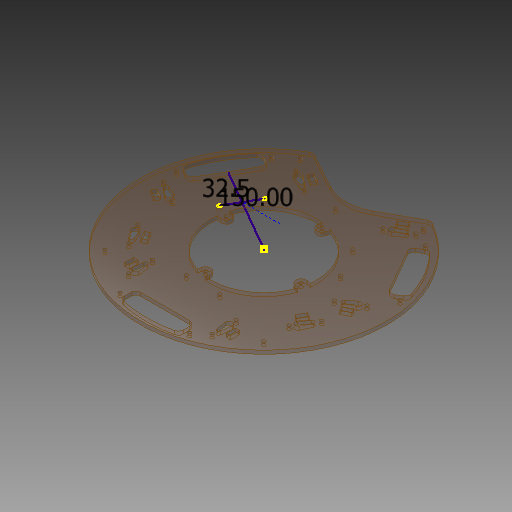
# Autodesk Inventor part: Base Plate
Saved by Autodesk Inventor 2018 (Build 220112000, 112)
## iProperties
Created: 2018-06-09
Part Number: Base Plate
Material: Polycarbonate, Smoke
Document SubType Name: Modeling
Designer: matth
Density: 1.2 g/cm^3
Appearance: Polycarbonate - Smoked
Mass: 68.8763 g
Surface Area: 521.491 cm^2
Volume: 68.8763 cm^3
Author: matth
Autodesk Inventor part; units mm, degrees
ref_plane "YZ Plane" through (0, 0, 0) normal (1, 0, 0) x (0, 1, 0)
ref_plane "XZ Plane" through (0, 0, 0) normal (0, 1, 0) x (-1, 0, 0)
ref_plane "XY Plane" through (0, 0, 0) normal (0, 0, 1) x (1, 0, 0)
sketch "Sketch1" plane through (0, 0, 0) normal (0, 1, 0) x (-1, 0, 0)
  circle A0 centre (0, 0) radius 105
  dimension "d0" = 210
  constraints: 1 centre point, 1 coincident
  measures "d0" diameter of A0
extrude "Blank Disk" add sketch "Sketch1" along normal blind 3
sketch "Sketch2" plane through (0, 3, 0) normal (0, 1, 0) x (1, 0, 0)
  line L0 (0, 0) -> (90.9327, 52.5)
  line L1 (0, 0) -> (105, 0) construction
  line L2 (0, 0) -> (-90.9327, 52.5)
  circle A0 centre (0, 0) radius 105 projected
  line L3 (0, 0) -> (0, -105)
  line L4 (90.9327, 52.5) -> (78.4327, 74.1506)
  line L5 (90.9327, 52.5) -> (103.4327, 30.8494)
  circle A1 centre (0, 0) radius 100
  line L6 (78.4327, 74.1506) -> (71.3525, 70.0629)
  line L7 (103.4327, 30.8494) -> (96.3525, 26.7617)
  line L8 (96.3525, 26.7617) -> (85.0942, 20.2617)
  line L9 (85.0942, 20.2617) -> (60.0942, 63.5629)
  line L10 (60.0942, 63.5629) -> (71.3525, 70.0629)
  arc A2 (96.3525, 26.7617) -> (71.3525, 70.0629) centre (0, 0) ccw
  line L11 (-90.9327, 52.5) -> (-78.4327, 74.1506)
  line L12 (-78.4327, 74.1506) -> (-103.4327, 30.8494)
  line L13 (-103.4327, 30.8494) -> (-96.3525, 26.7617)
  line L14 (-96.3525, 26.7617) -> (-85.0942, 20.2617)
  line L15 (-85.0942, 20.2617) -> (-60.0942, 63.5629)
  line L16 (-60.0942, 63.5629) -> (-71.3525, 70.0629)
  arc A3 (-71.3525, 70.0629) -> (-96.3525, 26.7617) centre (0, 0) ccw
  line L17 (0, -105) -> (25, -105)
  line L18 (25, -105) -> (25, -96.8246)
  line L19 (25, -96.8246) -> (25, -83.8246)
  line L20 (25, -83.8246) -> (-25, -83.8246)
  line L21 (-25, -83.8246) -> (-25, -96.8246)
  arc A4 (-25, -96.8246) -> (25, -96.8246) centre (0, 0) ccw
  dimension "d3" = 105
  dimension "d4" = 30
  dimension "d5" = 25
  dimension "d6" = 25
  dimension "d7" = 200
  dimension "d8" = 13
  dimension "d9" = 25
  dimension "d10" = 50
  dimension "d11" = 13
  dimension "d12" = 25
  dimension "d13" = 13
  dimension "d14" = 50
  constraints: 44 end point, 14 point on circle, 7 perpendicular, 5 point on line, 4 centre point, 2 concentric, 2 horizontal, 1 coincident, 1 equal length, 1 parallel, 1 vertical
  measures "d3" distance of L0.start L0.end
  measures "d4" angle of L1 L0
  measures "d5" distance of L0.end L4.end
  measures "d6" distance of L0.end L5.end
  measures "d7" diameter of A1
  measures "d8" distance of L7.end L8.end
  measures "d9" distance of L2.end L11.end
  measures "d10" distance of L11.end L12.end
  measures "d11" distance of L13.end L14.end
  measures "d12" distance of L3.end L17.end
  measures "d13" distance of L18.end L19.end
  measures "d14" distance of L19.end L20.end
extrude "Wheel Holes" cut sketch "Sketch2" against normal blind 3 contours L9 L10 A1 L0 | L0 A1 L8 L9 | L15 L14 A1 L2 | L2 A1 L16 L15 | L20 L19 A1 L3 | L3 A1 L21 L20
sketch "Sketch3" plane through (0, 3, 0) normal (0, 1, 0) x (1, 0, 0)
  line L0 (-60.0942, 63.5629) -> (-71.3525, 70.0629) projected
  line L1 (-96.3525, 26.7617) -> (-85.0942, 20.2617) projected
  line L2 (-71.3525, 70.0629) -> (-96.3525, 26.7617)
  line L3 (-83.8525, 48.4123) -> (-80.3884, 46.4123)
  line L4 (-80.3884, 46.4123) -> (-77.7904, 44.9123)
  line L5 (-77.7904, 44.9123) -> (-72.5942, 41.9123)
  line L6 (-72.5942, 41.9123) -> (-44.6649, 25.7873)
  line L7 (-60.0942, 63.5629) -> (-85.0942, 20.2617) projected
  line L8 (-72.5942, 41.9123) -> (-40.3442, 41.9123) construction
  line L9 (-44.6649, 25.7873) -> (-37.6149, 37.9983)
  line L10 (-37.6149, 37.9983) -> (-51.7149, 13.5763)
  circle A0 centre (-37.6149, 37.9983) radius 1.25
  circle A1 centre (-51.7149, 13.5763) radius 1.25
  line L11 (-72.5942, 41.9123) -> (-13.7045, 7.9123)
  line L12 (-13.7045, 7.9123) -> (-7.4545, 18.7376)
  line L13 (-13.7045, 7.9123) -> (-19.9545, -2.913)
  line L14 (85.0942, 20.2617) -> (60.0942, 63.5629) projected
  line L15 (72.5942, 41.9123) -> (44.6649, 25.7873)
  line L16 (72.5942, 41.9123) -> (104.8442, 41.9123) construction
  line L17 (44.6649, 25.7873) -> (37.6149, 37.9983)
  line L18 (37.6149, 37.9983) -> (51.7149, 13.5763)
  circle A2 centre (37.6149, 37.9983) radius 1.25
  circle A3 centre (51.7149, 13.5763) radius 1.25
  line L19 (25, -83.8246) -> (-25, -83.8246) projected
  line L20 (0, -83.8246) -> (0, -51.5746)
  line L21 (0, -51.5746) -> (14.1, -51.5746)
  line L22 (14.1, -51.5746) -> (-14.1, -51.5746)
  circle A4 centre (-14.1, -51.5746) radius 1.25
  circle A5 centre (14.1, -51.5746) radius 1.25
  point P0 (0, 0)
  dimension "d17" = 4
  dimension "d18" = 3
  dimension "d19" = 32.25
  dimension "d20" = 30
  dimension "d22" = 14.1
  dimension "d23" = 28.2
  dimension "d24" = 2.5
  dimension "d25" = 2.5
  dimension "d26" = 68
  dimension "d27" = 12.5
  dimension "d28" = 12.5
  dimension "d29" = 32.25
  dimension "d30" = 150
  dimension "d31" = 14.1
  dimension "d32" = 90
  dimension "d33" = 28.2
  dimension "d34" = 2.5
  dimension "d35" = 2.5
  dimension "d36" = 32.25
  dimension "d37" = 14.1
  dimension "d38" = 28.2
  dimension "d39" = 2.5
  dimension "d40" = 2.5
  constraints: 36 end point, 6 centre point, 6 coincident, 5 perpendicular, 5 point on line, 3 midpoint, 2 equal length, 2 horizontal, 1 parallel, 1 vertical
  measures "d17" distance of L3.start L3.end
  measures "d18" distance of L3.end L4.end
  measures "d19" distance of L5.end L6.end
  measures "d20" angle of L6 L8
  measures "d22" distance of L6.end L9.end
  measures "d23" distance of L9.end L10.end
  measures "d24" diameter of A0
  measures "d25" diameter of A1
  measures "d26" distance of L5.end L11.end
  measures "d27" distance of L11.end L12.end
  measures "d28" distance of L11.end L13.end
  measures "d29" distance of L15.start L15.end
  measures "d30" angle of L15 L16
  measures "d31" distance of L15.end L17.end
  measures "d32" angle of L15 L17
  measures "d33" distance of L17.end L18.end
  measures "d34" diameter of A2
  measures "d35" diameter of A3
  measures "d36" distance of L20.start L20.end
  measures "d37" distance of L20.end L21.end
  measures "d38" distance of L21.end L22.end
  measures "d39" diameter of A4
  measures "d40" diameter of A5
extrude "Motor Mount Holes" cut sketch "Sketch3" against normal blind 3 contours A0 | A1 | A2 | A3 | A4 | A5
sketch "Sketch5" plane through (0, 3, 0) normal (0, 1, 0) x (1, 0, 0)
  line L0 (0, 0) -> (40, 69.282)
  line L1 (0, 0) -> (80, 0) construction
  line L2 (0, 0) -> (80, 0)
  line L3 (0, 0) -> (69.282, -40)
  line L4 (0, 0) -> (80, 0) construction
  line L5 (0, 0) -> (40, -69.282)
  line L6 (0, 0) -> (80, 0) construction
  line L7 (0, 0) -> (-40, 69.282)
  line L8 (0, 0) -> (80, 0) construction
  line L9 (0, 0) -> (-80, 0)
  line L10 (0, 0) -> (-69.282, -40)
  line L11 (0, 0) -> (80, 0) construction
  line L12 (0, 0) -> (-40.0125, -69.3038)
  line L13 (-40, 69.282) -> (-32.301, 64.837)
  line L14 (-32.301, 64.837) -> (-27.3517, 61.9795)
  line L15 (-40, 69.282) -> (-44.9493, 72.1395)
  line L16 (-36.1505, 67.0595) -> (-33.293, 72.0089)
  line L17 (-36.1505, 67.0595) -> (-30.4355, 67.0595) construction
  line L18 (-33.293, 72.0089) -> (-29.9935, 70.1039)
  line L19 (-33.293, 72.0089) -> (-29.483, 72.0089) construction
  line L20 (-29.9935, 70.1039) -> (-28.0885, 73.4034)
  line L21 (-28.0885, 73.4034) -> (-34.6876, 77.2134)
  line L22 (-34.6876, 77.2134) -> (-36.5926, 73.9139)
  line L23 (-36.5926, 73.9139) -> (-33.293, 72.0089)
  circle A0 centre (-40, 69.282) radius 2.75
  circle A1 centre (-44.9493, 72.1395) radius 1.5
  circle A2 centre (-27.3517, 61.9795) radius 1.5
  circle A3 centre (-32.301, 64.837) radius 1.6
  line L24 (-40, 69.282) -> (-38.3069, 71.4491)
  line L25 (-40, 69.282) -> (-37.25, 69.282) construction
  line L26 (-40, 69.282) -> (-41.0302, 66.7323)
  line L27 (-40, 69.282) -> (-37.25, 69.282) construction
  line L28 (-32.301, 64.837) -> (-31.501, 66.2227)
  line L29 (-32.301, 64.837) -> (-30.701, 64.837) construction
  line L30 (-32.301, 64.837) -> (-33.101, 63.4514)
  line L31 (-33.101, 63.4514) -> (-41.0302, 66.7323)
  line L32 (-31.501, 66.2227) -> (-38.3069, 71.4491)
  line L33 (40, 69.282) -> (47.699, 73.727)
  line L34 (40, 69.282) -> (48.89, 69.282) construction
  line L35 (47.699, 73.727) -> (52.6483, 76.5845)
  line L36 (40, 69.282) -> (35.0507, 66.4245)
  line L37 (43.8495, 71.5045) -> (40.992, 76.4539)
  line L38 (40.992, 76.4539) -> (44.2915, 78.3589)
  line L39 (44.2915, 78.3589) -> (42.3865, 81.6584)
  line L40 (42.3865, 81.6584) -> (35.7874, 77.8484)
  line L41 (35.7874, 77.8484) -> (37.6924, 74.5489)
  line L42 (37.6924, 74.5489) -> (40.992, 76.4539)
  circle A4 centre (40, 69.282) radius 2.75
  circle A5 centre (47.699, 73.727) radius 1.6
  circle A6 centre (52.6483, 76.5845) radius 1.5
  circle A7 centre (35.0507, 66.4245) radius 1.5
  line L43 (40, 69.282) -> (38.9698, 71.8318)
  line L44 (40, 69.282) -> (42.75, 69.282) construction
  line L45 (40, 69.282) -> (41.6931, 67.115)
  line L46 (40, 69.282) -> (42.75, 69.282) construction
  line L47 (47.699, 73.727) -> (46.899, 75.1127)
  line L48 (47.699, 73.727) -> (49.299, 73.727) construction
  line L49 (46.899, 75.1127) -> (48.499, 72.3414)
  line L50 (48.499, 72.3414) -> (41.6931, 67.115)
  line L51 (38.9698, 71.8318) -> (46.899, 75.1127)
  line L52 (80, 0) -> (72.336, -4.5051)
  line L53 (72.336, -4.5051) -> (67.4092, -7.4012)
  line L54 (80, 0) -> (84.9493, 2.8575)
  circle A8 centre (80, 0) radius 2.75
  circle A9 centre (84.9493, 2.8575) radius 1.5
  circle A10 centre (72.336, -4.5051) radius 1.6
  circle A11 centre (67.4092, -7.4012) radius 1.5
  line L55 (76.168, -2.2525) -> (78.7862, -7.3325)
  line L56 (78.7862, -7.3325) -> (82.1729, -5.5871)
  line L57 (82.1729, -5.5871) -> (83.9183, -8.9738)
  line L58 (83.9183, -8.9738) -> (77.145, -12.4646)
  line L59 (77.145, -12.4646) -> (75.3995, -9.078)
  line L60 (75.3995, -9.078) -> (78.7862, -7.3325)
  line L61 (80, 0) -> (78.3069, 2.167)
  line L62 (80, 0) -> (82.75, 0) construction
  line L63 (80, 0) -> (81.0302, -2.5498)
  line L64 (72.336, -4.5051) -> (71.5528, -3.1099)
  line L65 (72.336, -4.5051) -> (73.1193, -5.9002)
  line L66 (73.1193, -5.9002) -> (81.0302, -2.5498)
  line L67 (71.5528, -3.1099) -> (78.3069, 2.167)
  line L68 (40, -69.282) -> (40, -78.172)
  line L69 (40, -78.172) -> (40, -83.887)
  line L70 (40, -69.282) -> (40, -63.567)
  line L71 (40, -73.727) -> (45.715, -73.727)
  line L72 (45.715, -73.727) -> (45.715, -69.917)
  line L73 (45.715, -69.917) -> (49.525, -69.917)
  line L74 (49.525, -69.917) -> (49.525, -77.537)
  line L75 (49.525, -77.537) -> (45.715, -77.537)
  line L76 (45.715, -77.537) -> (45.715, -73.727)
  circle A12 centre (40, -63.567) radius 1.5
  circle A13 centre (40, -83.887) radius 1.5
  circle A14 centre (40, -78.172) radius 1.6
  circle A15 centre (40, -69.282) radius 2.75
  line L77 (40, -69.282) -> (42.7232, -69.6648)
  line L78 (40, -69.282) -> (42.75, -69.282) construction
  line L79 (42.7232, -69.6648) -> (37.2768, -69.6648)
  line L80 (40, -78.172) -> (41.6, -78.172)
  line L81 (40, -78.172) -> (38.4, -78.172)
  line L82 (38.4, -78.172) -> (37.2768, -69.6648)
  line L83 (41.6, -78.172) -> (42.7232, -69.6648)
  line L84 (69.282, -40) -> (73.936, -32.4255)
  line L85 (73.936, -32.4255) -> (76.9279, -27.5562)
  line L86 (69.282, -40) -> (66.4245, -44.9493)
  line L87 (71.609, -36.2128) -> (66.6597, -33.3553)
  line L88 (66.6597, -33.3553) -> (68.5647, -30.0557)
  line L89 (68.5647, -30.0557) -> (65.2651, -28.1507)
  line L90 (65.2651, -28.1507) -> (61.4551, -34.7498)
  line L91 (61.4551, -34.7498) -> (64.7547, -36.6548)
  line L92 (64.7547, -36.6548) -> (66.6597, -33.3553)
  circle A16 centre (76.9279, -27.5562) radius 1.5
  circle A17 centre (66.4245, -44.9493) radius 1.5
  circle A18 centre (69.282, -40) radius 2.75
  circle A19 centre (73.936, -32.4255) radius 1.6
  line L93 (-40.0125, -69.3038) -> (-40.0125, -60.4138)
  line L94 (-40.0125, -60.4138) -> (-40.0125, -54.6988)
  line L95 (-40.0125, -69.3038) -> (-40.0125, -75.0188)
  line L96 (-40.0125, -64.8588) -> (-45.7275, -64.8588)
  line L97 (-45.7275, -64.8588) -> (-45.7275, -61.0488)
  line L98 (-45.7275, -61.0488) -> (-49.5375, -61.0488)
  line L99 (-49.5375, -61.0488) -> (-49.5375, -68.6688)
  line L100 (-49.5375, -68.6688) -> (-45.7275, -68.6688)
  line L101 (-45.7275, -68.6688) -> (-45.7275, -64.8588)
  circle A20 centre (-40.0125, -69.3038) radius 2.75
  circle A21 centre (-40.0125, -60.4138) radius 1.6
  circle A22 centre (-40.0125, -54.6988) radius 1.5
  circle A23 centre (-40.0125, -75.0188) radius 1.5
  line L102 (-69.282, -40) -> (-64.837, -47.699)
  line L103 (-64.837, -47.699) -> (-61.9795, -52.6483)
  line L104 (-69.282, -40) -> (-72.1395, -35.0507)
  line L105 (-67.0595, -43.8495) -> (-62.1102, -40.992)
  line L106 (-67.0595, -43.8495) -> (-61.3445, -43.8495) construction
  line L107 (-62.1102, -40.992) -> (-60.2052, -44.2915)
  line L108 (-60.2052, -44.2915) -> (-56.9056, -42.3865)
  line L109 (-56.9056, -42.3865) -> (-60.7156, -35.7874)
  line L110 (-60.7156, -35.7874) -> (-64.0152, -37.6924)
  line L111 (-64.0152, -37.6924) -> (-62.1102, -40.992)
  circle A24 centre (-69.282, -40) radius 2.75
  circle A25 centre (-72.1395, -35.0507) radius 1.5
  circle A26 centre (-64.837, -47.699) radius 1.6
  circle A27 centre (-61.9795, -52.6483) radius 1.5
  line L112 (-80, 0) -> (-87.699, 4.445)
  line L113 (-80, 0) -> (-71.11, 0) construction
  line L114 (-87.699, 4.445) -> (-92.6483, 7.3025)
  line L115 (-80, 0) -> (-75.0507, -2.8575)
  line L116 (-80, 0) -> (-74.285, 0) construction
  line L117 (-83.8495, 2.2225) -> (-86.707, -2.7268)
  line L118 (-83.8495, 2.2225) -> (-78.1345, 2.2225) construction
  line L119 (-86.707, -2.7268) -> (-90.0065, -0.8218)
  line L120 (-90.0065, -0.8218) -> (-91.9115, -4.1214)
  line L121 (-91.9115, -4.1214) -> (-85.3124, -7.9314)
  line L122 (-85.3124, -7.9314) -> (-83.4074, -4.6318)
  line L123 (-83.4074, -4.6318) -> (-86.707, -2.7268)
  circle A28 centre (-80, 0) radius 2.75
  circle A29 centre (-87.699, 4.445) radius 1.6
  circle A30 centre (-92.6483, 7.3025) radius 1.5
  circle A31 centre (-75.0507, -2.8575) radius 1.5
  line L124 (69.282, -40) -> (67.115, -38.3069)
  line L125 (69.282, -40) -> (72.032, -40) construction
  line L126 (69.282, -40) -> (71.8318, -41.0302)
  line L127 (69.282, -40) -> (72.032, -40) construction
  line L128 (73.936, -32.4255) -> (72.5504, -31.6255)
  line L129 (73.936, -32.4255) -> (75.536, -32.4255) construction
  line L130 (72.5504, -31.6255) -> (75.3217, -33.2255)
  line L131 (71.8318, -41.0302) -> (75.3217, -33.2255)
  line L132 (67.115, -38.3069) -> (72.5504, -31.6255)
  line L133 (-40.0125, -69.3038) -> (-37.2893, -68.921)
  line L134 (-40.0125, -69.3038) -> (-37.2625, -69.3038) construction
  line L135 (-40.0125, -69.3038) -> (-42.7389, -68.9438)
  line L136 (-40.0125, -60.4138) -> (-41.6125, -60.4138)
  line L137 (-41.6125, -60.4138) -> (-38.4125, -60.4138)
  line L138 (-37.2893, -68.921) -> (-38.4125, -60.4138)
  line L139 (-42.7389, -68.9438) -> (-41.6125, -60.4138)
  line L140 (-69.282, -40) -> (-66.7323, -38.9698)
  line L141 (-69.282, -40) -> (-71.4491, -41.6931)
  line L142 (-64.837, -47.699) -> (-63.4514, -46.899)
  line L143 (-63.4514, -46.899) -> (-66.2227, -48.499)
  line L144 (-63.4514, -46.899) -> (-66.7323, -38.9698)
  line L145 (-66.2227, -48.499) -> (-71.4491, -41.6931)
  line L146 (-80, 0) -> (-78.9698, 2.5498)
  line L147 (-80, 0) -> (-77.25, 0) construction
  line L148 (-80, 0) -> (-81.6931, -2.167)
  line L149 (-87.699, 4.445) -> (-86.899, 5.8306)
  line L150 (-87.699, 4.445) -> (-88.499, 3.0594)
  line L151 (-86.899, 5.8306) -> (-78.9698, 2.5498)
  line L152 (-81.6931, -2.167) -> (-88.499, 3.0594)
  dimension "d157" = 3.2
  dimension "d108" = 80
  dimension "d109" = 60
  dimension "d110" = 80
  dimension "d111" = 80
  dimension "d112" = 30
  dimension "d113" = 80
  dimension "d114" = 60
  dimension "d115" = 80
  dimension "d116" = 120
  dimension "d117" = 80
  dimension "d118" = 80
  dimension "d119" = 150
  dimension "d120" = 8.89
  dimension "d121" = 5.715
  dimension "d122" = 5.715
  dimension "d123" = 5.715
  dimension "d124" = 60
  dimension "d125" = 3.81
  dimension "d126" = 30
  dimension "d127" = 3.81
  dimension "d128" = 7.62
  dimension "d129" = 5.5
  dimension "d130" = 3
  dimension "d131" = 3
  dimension "d132" = 3.2
  dimension "d133" = 52
  dimension "d134" = 112
  dimension "d135" = 60
  dimension "d148" = 8.89
  dimension "d149" = 30
  dimension "d150" = 5.715
  dimension "d151" = 5.715
  dimension "d152" = 5.715
  dimension "d153" = 3.81
  dimension "d154" = 3.81
  dimension "d155" = 7.62
  dimension "d156" = 5.5
  dimension "d158" = 3
  dimension "d159" = 3
  dimension "d160" = 112
  dimension "d161" = 52
  dimension "d162" = 1.6
  dimension "d163" = 120
  dimension "d164" = 8.89
  dimension "d165" = 5.715
  dimension "d166" = 5.715
  dimension "d167" = 5.5
  dimension "d168" = 3
  dimension "d169" = 3.2
  dimension "d170" = 3
  dimension "d171" = 5.715
  dimension "d172" = 3.81
  dimension "d173" = 3.81
  dimension "d174" = 7.62
  dimension "d175" = 128
  dimension "d176" = 8.89
  dimension "d177" = 5.715
  dimension "d178" = 5.715
  dimension "d179" = 5.715
  dimension "d180" = 3.81
  dimension "d181" = 3.81
  dimension "d182" = 7.62
  dimension "d183" = 3
  dimension "d184" = 3
  constraints: 306 end point, 40 perpendicular, 32 coincident, 31 centre point, 30 horizontal, 30 point on circle, 25 equal length, 23 point on line, 8 midpoint, 4 vertical, 1 collinear, 1 parallel, 1 tangent, 3 other
  measures "d108" distance of L0.start L0.end
  measures "d109" angle of L1 L0
  measures "d110" distance of L0.start L1.end
  measures "d111" distance of L0.start L3.end
  measures "d112" angle of L3 L4
  measures "d113" distance of L0.start L5.end
  measures "d114" angle of L5 L6
  measures "d115" distance of L0.start L7.end
  measures "d116" angle of L8 L7
  measures "d117" distance of L0.start L9.end
  measures "d118" distance of L0.start L10.end
  measures "d119" angle of L10 L11
  measures "d120" distance of L7.end L13.end
  measures "d121" distance of L13.end L14.end
  measures "d122" distance of L15.start L15.end
  measures "d123" distance of L16.start L16.end
  measures "d124" angle of L17 L16
  measures "d125" distance of L16.end L18.end
  measures "d126" angle of L18 L19
  measures "d127" distance of L18.end L20.end
  measures "d128" distance of L20.end L21.end
  measures "d129" diameter of A0
  measures "d130" diameter of A1
  measures "d131" diameter of A2
  measures "d132" diameter of A3
  measures "d133" angle of L25 L24
  measures "d134" angle of L26 L27
  measures "d135" angle of L29 L28
  measures "d148" distance of L0.end L33.end
  measures "d149" angle of L34 L33
  measures "d150" distance of L33.end L35.end
  measures "d151" distance of L0.end L36.end
  measures "d152" distance of L37.start L37.end
  measures "d153" distance of L37.end L38.end
  measures "d154" distance of L38.end L39.end
  measures "d155" distance of L39.end L40.end
  measures "d156" diameter of A4
  measures "d158" diameter of A6
  measures "d159" diameter of A7
  measures "d160" angle of L44 L43
  measures "d161" angle of L45 L46
  measures "d162" distance of L47.start L47.end
  measures "d163" angle of L48 L47
  measures "d164" distance of L11.end L52.end
  measures "d165" distance of L52.end L53.end
  measures "d166" distance of L11.end L54.end
  measures "d167" diameter of A8
  measures "d168" diameter of A9
  measures "d169" diameter of A10
  measures "d170" diameter of A11
  measures "d171" distance of L55.start L55.end
  measures "d172" distance of L55.end L56.end
  measures "d173" distance of L56.end L57.end
  measures "d174" distance of L57.end L58.end
  measures "d175" angle of L62 L61
  measures "d176" distance of L5.end L68.end
  measures "d177" distance of L68.end L69.end
  measures "d178" distance of L5.end L70.end
  measures "d179" distance of L71.start L71.end
  measures "d180" distance of L71.end L72.end
  measures "d181" distance of L72.end L73.end
  measures "d182" distance of L73.end L74.end
  measures "d183" diameter of A12
  measures "d184" diameter of A13
extrude "Outer Light Sensors" cut sketch "Sketch5" against normal blind 3
sketch "Sketch6" plane through (0, 3, 0) normal (0, 1, 0) x (1, 0, 0)
  line L0 (-50, 92.3309) -> (50, 92.3309)
  line L1 (0, 92.3309) -> (0, 64.8309)
  line L2 (0, 64.8309) -> (50, 92.3309)
  line L3 (-50, 92.3309) -> (0, 64.8309)
  arc A0 (50, 92.3309) -> (-50, 92.3309) centre (0, 0) ccw
  point P0 (0, 0)
  dimension "d245" = 27.5
  constraints: 8 end point, 2 point on circle, 1 centre point, 1 midpoint, 1 vertical
  measures "d245" distance of L1.start L1.end
extrude "Capture Zone Cutout" cut sketch "Sketch6" against normal blind 3
fillet "Capture Zone Curve" radius 37 1 edges at (0, 1.5, -64.8309)
sketch "Sketch7" plane through (0, 3, 0) normal (0, 1, 0) x (1, 0, 0)
  arc A0 (-71.3525, 70.0629) -> (-96.3525, 26.7617) centre (0, 0) ccw projected
  line L0 (-71.3525, 70.0629) -> (-67.8884, 68.0629)
  line L1 (-60.0942, 63.5629) -> (-71.3525, 70.0629) projected
  line L2 (-67.8884, 68.0629) -> (-65.6389, 71.9592)
  circle A1 centre (-65.6389, 71.9592) radius 1.5
  line L3 (-96.3525, 26.7617) -> (-92.8884, 24.7617)
  line L4 (-96.3525, 26.7617) -> (-85.0942, 20.2617) projected
  line L5 (-92.8884, 24.7617) -> (-95.1379, 20.8654)
  circle A2 centre (-95.1379, 20.8654) radius 1.5
  line L6 (71.3525, 70.0629) -> (67.8884, 68.0629)
  line L7 (71.3525, 70.0629) -> (60.0942, 63.5629) projected
  line L8 (67.8884, 68.0629) -> (65.6389, 71.9592)
  line L9 (85.0942, 20.2617) -> (96.3525, 26.7617) projected
  line L10 (96.3525, 26.7617) -> (92.8884, 24.7617)
  line L11 (92.8884, 24.7617) -> (95.1379, 20.8654)
  circle A3 centre (95.1379, 20.8654) radius 1.5
  circle A4 centre (65.6389, 71.9592) radius 1.5
  line L12 (-25, -83.8246) -> (-25, -96.8246) projected
  line L13 (-25, -96.8246) -> (-25, -92.8246)
  line L14 (-25, -92.8246) -> (-29.499, -92.8246)
  line L15 (25, -96.8246) -> (25, -83.8246) projected
  line L16 (25, -96.8246) -> (25, -92.8246)
  line L17 (25, -92.8246) -> (29.499, -92.8246)
  circle A5 centre (-29.499, -92.8246) radius 1.5
  circle A6 centre (29.499, -92.8246) radius 1.5
  point P0 (0, 0)
  dimension "d249" = 4
  dimension "d250" = 4.499
  dimension "d251" = 3
  dimension "d252" = 4
  dimension "d253" = 4.499
  dimension "d254" = 3
  dimension "d255" = 4
  dimension "d256" = 4.499
  dimension "d257" = 4
  dimension "d258" = 4.499
  dimension "d259" = 3
  dimension "d260" = 3
  dimension "d261" = 4
  dimension "d262" = 4.499
  dimension "d263" = 4
  dimension "d264" = 4.499
  dimension "d265" = 3
  dimension "d266" = 3
  constraints: 24 end point, 6 centre point, 6 coincident, 6 perpendicular, 6 point on line
  measures "d249" distance of L0.start L0.end
  measures "d250" distance of L0.end L2.end
  measures "d251" diameter of A1
  measures "d252" distance of L3.start L3.end
  measures "d253" distance of L3.end L5.end
  measures "d254" diameter of A2
  measures "d255" distance of L6.start L6.end
  measures "d256" distance of L6.end L8.end
  measures "d257" distance of L9.end L10.end
  measures "d258" distance of L10.end L11.end
  measures "d259" diameter of A3
  measures "d260" diameter of A4
  measures "d261" distance of L12.end L13.end
  measures "d262" distance of L13.end L14.end
  measures "d263" distance of L15.start L16.end
  measures "d264" distance of L16.end L17.end
  measures "d265" diameter of A5
  measures "d266" diameter of A6
extrude "Wheel Guard Mounting Holes" cut sketch "Sketch7" against normal blind 3
sketch "Sketch9" plane through (0, 3, 0) normal (0, 1, 0) x (1, 0, 0)
  line L0 (0, 0) -> (93.6948, -25.1054)
  line L1 (0, 0) -> (97, 0) construction
  line L2 (0, 0) -> (-93.6948, -25.1054)
  line L3 (0, 0) -> (97, 0) construction
  circle A0 centre (-93.6948, -25.1054) radius 1.5
  circle A1 centre (93.6948, -25.1054) radius 1.5
  dimension "d290" = 97
  dimension "d291" = 15
  dimension "d292" = 97
  dimension "d293" = 165
  dimension "d294" = 3
  dimension "d295" = 3
  constraints: 8 end point, 2 centre point, 2 coincident, 2 equal length, 2 horizontal
  measures "d290" distance of L0.start L0.end
  measures "d291" angle of L0 L1
  measures "d292" distance of L0.start L2.end
  measures "d293" angle of L2 L3
  measures "d294" diameter of A0
  measures "d295" diameter of A1
extrude "Standoff Holes" cut sketch "Sketch9" against normal blind 3
fillet "Capture Zone and Wheel Guard Fillets" radius 4 14 edges at (-71.3525, 1.5, -70.0629) (-60.0942, 1.5, -63.5629) (-85.0942, 1.5, -20.2617) (-96.3525, 1.5, -26.7617) (-25, 1.5, 83.8246) (-25, 1.5, 96.8246) (25, 1.5, 83.8246) (25, 1.5, 96.8246) (85.0942, 1.5, -20.2617) (96.3525, 1.5, -26.7617) (71.3525, 1.5, -70.0629) (60.0942, 1.5, -63.5629) (50, 1.5, -92.3309) (-50, 1.5, -92.3309)
sketch "Sketch13" plane through (0, 3, 0) normal (0, 1, 0) x (1, 0, 0)
  circle A0 centre (0, 0) radius 45
  line L0 (0, 45) -> (0, 51)
  line L1 (0, 0) -> (44.1673, -25.5)
  line L2 (0, 0) -> (51, 0) construction
  line L3 (0, 0) -> (-44.1673, -25.5)
  line L4 (0, 0) -> (51, 0) construction
  circle A1 centre (-44.1673, -25.5) radius 1.5
  circle A2 centre (44.1673, -25.5) radius 1.5
  circle A3 centre (0, 51) radius 1.5
  dimension "d380" = 90
  dimension "d381" = 6
  dimension "d382" = 51
  dimension "d383" = 30
  dimension "d384" = 51
  dimension "d385" = 150
  dimension "d386" = 3
  dimension "d387" = 3
  dimension "d388" = 3
  constraints: 10 end point, 4 coincident, 3 centre point, 2 equal length, 2 horizontal, 1 vertical, 1 vertical alignment, 2 other
  measures "d381" distance of L0.start L0.end
  measures "d382" distance of L1.start L1.end
  measures "d383" angle of L1 L2
  measures "d384" distance of L1.start L3.end
  measures "d385" angle of L3 L4
  measures "d386" diameter of A1
  measures "d387" diameter of A2
  measures "d388" diameter of A3
extrude "Main Light Sensor PCB Hole" cut sketch "Sketch13" against normal blind 3
sketch "Sketch19" plane through (0, 3, 0) normal (0, 1, 0) x (1, 0, 0)
  arc A0 (-17.831, 74.638) -> (17.831, 74.638) centre (0, 107.058) ccw projected
  line L0 (0, 70.058) -> (0, 61.058)
  line L1 (-17.831, 74.638) -> (-48.0629, 91.2655) projected
  line L2 (-48.0629, 91.2655) -> (-40.177, 86.9283)
  line L3 (-48.0629, 91.2655) -> (-52.4002, 83.3796)
  line L4 (48.0629, 91.2655) -> (17.831, 74.638) projected
  line L5 (48.0629, 91.2655) -> (40.177, 86.9283)
  line L6 (48.0629, 91.2655) -> (52.4002, 83.3796)
  circle A1 centre (52.4002, 83.3796) radius 1.5
  circle A2 centre (0, 61.058) radius 1.5
  circle A3 centre (-52.4002, 83.3796) radius 1.5
  point P0 (0, 0)
  dimension "d405" = 9
  dimension "d406" = 9
  dimension "d407" = 9
  dimension "d408" = 9
  dimension "d409" = 9
  dimension "d410" = 3
  dimension "d411" = 3
  dimension "d412" = 3
  constraints: 10 end point, 3 centre point, 3 coincident, 2 point on line, 1 perpendicular, 1 point on circle, 1 vertical
  measures "d405" distance of L0.start L0.end
  measures "d406" distance of L1.end L2.end
  measures "d407" distance of L1.end L3.end
  measures "d408" distance of L4.start L5.end
  measures "d409" distance of L4.start L6.end
  measures "d410" diameter of A1
  measures "d411" diameter of A2
  measures "d412" diameter of A3
extrude "Extrusion13" cut sketch "Sketch19" against normal blind 10
sketch "Sketch22" plane through (0, 0, 0) normal (0, -1, 0) x (1, 0, 0)
  circle A0 centre (-14.1, 51.5746) radius 1.25 projected
  circle A1 centre (14.1, 51.5746) radius 1.25 projected
  line L0 (-14.1, 51.5746) -> (14.1, 51.5746)
  line L1 (0, 51.5746) -> (0, 83.8246)
  line L2 (21, 83.8246) -> (-21, 83.8246) projected
  line L3 (-25, 87.8246) -> (-25, 93.675) projected
  line L4 (-25, 90.7498) -> (25, 90.7498)
  line L5 (25, 93.675) -> (25, 87.8246) projected
  line L6 (0, 83.8246) -> (0, 90.7498)
  line L7 (-2.9396, 90.7498) -> (-2.9396, 83.2498)
  line L8 (-2.9396, 83.2498) -> (-2.9396, 51.5746)
  circle A2 centre (-44.1673, 25.5) radius 1.5 projected
  circle A3 centre (-44.1673, 25.5) radius 1.5
  circle A4 centre (44.1673, 25.5) radius 1.5 projected
  circle A5 centre (44.1673, 25.5) radius 1.5
  circle A6 centre (0, -51) radius 1.5 projected
  circle A7 centre (0, -51) radius 1.5
  point P0 (0, 0)
  dimension "d416" = 6.9252
  dimension "d417" = 50
  dimension "d418" = 32.25
  dimension "d419" = 28.2
  dimension "d420" = 7.5
  dimension "d421" = 31.6752
  constraints: 12 end point, 5 midpoint, 3 centre point, 3 coincident, 3 point on line, 1 horizontal, 1 vertical
  measures "d416" distance of L1.end L6.end
  measures "d417" distance of L4.start L4.end
  measures "d418" distance of L1.start L1.end
  measures "d419" distance of L0.start L0.end
  measures "d420" distance of L7.start L7.end
  measures "d421" distance of L7.end L8.end
extrude "Extrusion14" add sketch "Sketch22" against normal blind 3 contours A2 | A4 | A6
sketch "Sketch23" plane through (0, 0, 0) normal (0, -1, 0) x (1, 0, 0)
  circle A0 centre (-14.1, 51.5746) radius 1.25 projected
  circle A1 centre (-14.1, 51.5746) radius 1.5
  circle A2 centre (14.1, 51.5746) radius 1.25 projected
  circle A3 centre (14.1, 51.5746) radius 1.5
  circle A4 centre (51.7149, -13.5763) radius 1.25 projected
  circle A5 centre (51.7149, -13.5763) radius 1.5
  circle A6 centre (37.6149, -37.9983) radius 1.25 projected
  circle A7 centre (37.6149, -37.9983) radius 1.5
  circle A8 centre (-37.6149, -37.9983) radius 1.25 projected
  circle A9 centre (-37.6149, -37.9983) radius 1.5
  circle A10 centre (-51.7149, -13.5763) radius 1.25 projected
  circle A11 centre (-51.7149, -13.5763) radius 1.5
  point P0 (0, 0)
  dimension "d424" = 3
  dimension "d425" = 3
  dimension "d426" = 3
  dimension "d427" = 3
  dimension "d428" = 3
  dimension "d429" = 3
  constraints: 6 centre point, 6 coincident
  measures "d424" diameter of A1
  measures "d425" diameter of A3
  measures "d426" diameter of A5
  measures "d427" diameter of A7
  measures "d428" diameter of A9
  measures "d429" diameter of A11
extrude "Extrusion15" cut sketch "Sketch23" against normal blind 3 contours A1 | A3 | A4 | A5 | A7 | A9 | A11
sketch "Sketch24" plane through (0, 0, 0) normal (0, -1, 0) x (1, 0, 0)
  line L0 (0, 0) -> (0, -40.64)
  line L1 (0, 0) -> (-40.64, 0)
  line L2 (0, 0) -> (0, 40.64)
  line L3 (0, 0) -> (40.64, 0)
  line L4 (0, -40.64) -> (-8.89, -40.64)
  line L5 (-40.64, 0) -> (-40.64, 8.89)
  line L6 (0, 40.64) -> (8.89, 40.64)
  line L7 (40.64, 0) -> (40.64, -8.89)
  circle A0 centre (40.64, -8.89) radius 4.5
  circle A1 centre (-8.89, -40.64) radius 4.5
  circle A2 centre (-40.64, 8.89) radius 4.5
  circle A3 centre (8.89, 40.64) radius 4.5
  line L8 (0, 0) -> (40.64, -8.89)
  line L9 (40.64, -8.89) -> (39.6784, -13.2861)
  line L10 (39.6784, -13.2861) -> (46.8912, -14.8638)
  line L11 (46.8912, -14.8638) -> (48.8144, -6.0717)
  line L12 (48.8144, -6.0717) -> (41.6016, -4.4939)
  line L13 (0, 0) -> (-8.89, -40.64)
  line L14 (0, 0) -> (-40.64, 8.89)
  line L15 (0, 0) -> (8.89, 40.64)
  line L16 (-8.89, -40.64) -> (-13.2861, -39.6784)
  line L17 (-13.2861, -39.6784) -> (-14.7969, -46.585)
  line L18 (-14.7969, -46.585) -> (-6.0048, -48.5083)
  line L19 (-6.0048, -48.5083) -> (-4.4939, -41.6016)
  line L20 (-4.4939, -41.6016) -> (-8.89, -40.64)
  line L21 (-40.64, 8.89) -> (-39.6784, 13.2861)
  line L22 (-39.6784, 13.2861) -> (-46.2908, 14.7325)
  line L23 (-46.2908, 14.7325) -> (-48.2141, 5.9404)
  line L24 (-48.2141, 5.9404) -> (-41.6016, 4.4939)
  line L25 (-40.64, 8.89) -> (-41.6016, 4.4939)
  line L26 (8.89, 40.64) -> (13.2861, 39.6784)
  line L27 (13.2861, 39.6784) -> (14.6704, 46.0066)
  line L28 (14.6704, 46.0066) -> (5.8783, 47.9299)
  line L29 (5.8783, 47.9299) -> (4.4939, 41.6016)
  circle A4 centre (8.89, -40.64) radius 4.5
  line L30 (13.2861, -39.6784) -> (14.7969, -46.585)
  line L31 (14.7969, -46.585) -> (6.0048, -48.5083)
  line L32 (6.0048, -48.5083) -> (4.4939, -41.6016)
  circle A5 centre (-40.64, -8.89) radius 4.5
  line L33 (-39.6784, -13.2861) -> (-46.2908, -14.7325)
  line L34 (-46.2908, -14.7325) -> (-48.2141, -5.9404)
  line L35 (-48.2141, -5.9404) -> (-41.6016, -4.4939)
  circle A6 centre (-8.89, 40.64) radius 4.5
  line L36 (-13.2861, 39.6784) -> (-14.6704, 46.0066)
  line L37 (-14.6704, 46.0066) -> (-5.8783, 47.9299)
  line L38 (-5.8783, 47.9299) -> (-4.4939, 41.6016)
  circle A7 centre (40.64, 8.89) radius 4.5
  line L39 (39.6784, 13.2861) -> (46.8912, 14.8638)
  line L40 (46.8912, 14.8638) -> (48.8144, 6.0717)
  line L41 (48.8144, 6.0717) -> (41.6016, 4.4939)
  dimension "d432" = 40.64
  dimension "d433" = 40.64
  dimension "d434" = 40.64
  dimension "d435" = 40.64
  dimension "d436" = 8.89
  dimension "d437" = 8.89
  dimension "d438" = 8.89
  dimension "d439" = 8.89
  dimension "d440" = 9
  dimension "d441" = 9
  dimension "d442" = 9
  dimension "d443" = 9
  dimension "d444" = 9
  dimension "d445" = 9
  constraints: 84 end point, 20 symmetric about line, 16 point on circle, 11 perpendicular, 8 centre point, 7 point on line, 4 coincident, 4 horizontal, 4 vertical, 1 tangent, 4 other
  measures "d432" distance of L0.start L0.end
  measures "d433" distance of L0.start L1.end
  measures "d434" distance of L0.start L2.end
  measures "d435" distance of L0.start L3.end
  measures "d436" distance of L0.end L4.end
  measures "d437" distance of L1.end L5.end
  measures "d438" distance of L2.end L6.end
  measures "d439" distance of L3.end L7.end
  measures "d440" diameter of A0
  measures "d441" diameter of A1
  measures "d442" diameter of A2
  measures "d443" diameter of A3
  measures "d444" distance of L10.end L11.end
  measures "d445" distance of L17.end L18.end
extrude "Extrusion16" cut sketch "Sketch24" along normal blind 3 contours L8 L9 A0 | A0 L7 L8 | L13 L16 A1 | A1 L4 L13 | L14 L21 A2 | A2 L5 L14 | L15 L26 A3 | A3 L6 L15 | A1 L20 L4 | A2 L25 L5 | A3 L26 L6 | A0 L9 L7 | A0 L12 L11 L10 | L16 L20 A1 | A1 L19 L18 L17 | L25 A2 L21 | A3 L29 L28 L27 | L24 L23 L22 A2
sketch "Sketch25" plane through (0, 0, 0) normal (0, -1, 0) x (1, 0, 0)
  arc A0 (-41.6016, 4.4939) -> (-39.6784, 13.2861) centre (-40.64, 8.89) ccw projected
  circle A1 centre (-40.64, 8.89) radius 1.5
  arc A2 (4.4939, 41.6016) -> (13.2861, 39.6784) centre (8.89, 40.64) ccw projected
  circle A3 centre (8.89, 40.64) radius 1.5
  arc A4 (41.6016, -4.4939) -> (39.6784, -13.2861) centre (40.64, -8.89) ccw projected
  circle A5 centre (40.64, -8.89) radius 1.5
  arc A6 (-4.4939, -41.6016) -> (-13.2861, -39.6784) centre (-8.89, -40.64) ccw projected
  circle A7 centre (-8.89, -40.64) radius 1.5
  point P0 (0, 0)
  dimension "d448" = 3
  dimension "d449" = 3
  dimension "d450" = 3
  dimension "d451" = 3
  constraints: 4 centre point, 4 coincident
  measures "d448" diameter of A1
  measures "d449" diameter of A3
  measures "d450" diameter of A5
  measures "d451" diameter of A7
extrude "Extrusion17" cut sketch "Sketch25" against normal blind 3
extrude "Extrusion18" add sketch "Sketch24" against normal blind 3 contours A4 | A4 L30 L31 L32 | A5 | A5 L33 L34 L35 | A6 | A6 L36 L37 L38 | A7 | A7 L39 L40 L41
sketch "Sketch26" plane through (0, 3, 0) normal (0, 1, 0) x (1, 0, 0)
  arc A0 (4.4939, 41.6016) -> (13.2861, 39.6784) centre (8.89, 40.64) ccw projected
  circle A1 centre (8.89, 40.64) radius 1.5
  arc A2 (-41.6016, 4.4939) -> (-39.6784, 13.2861) centre (-40.64, 8.89) ccw projected
  circle A3 centre (-40.64, 8.89) radius 1.5
  arc A4 (41.6016, -4.4939) -> (39.6784, -13.2861) centre (40.64, -8.89) ccw projected
  circle A5 centre (40.64, -8.89) radius 1.5
  arc A6 (-4.4939, -41.6016) -> (-13.2861, -39.6784) centre (-8.89, -40.64) ccw projected
  circle A7 centre (-8.89, -40.64) radius 1.5
  point P0 (0, 0)
  dimension "d456" = 3
  dimension "d457" = 3
  dimension "d458" = 3
  dimension "d459" = 3
  constraints: 4 centre point, 4 coincident
  measures "d456" diameter of A1
  measures "d457" diameter of A3
  measures "d458" diameter of A5
  measures "d459" diameter of A7
extrude "Extrusion19" cut sketch "Sketch26" against normal blind 3
sketch "Sketch28" plane through (0, 3, 0) normal (0, 1, 0) x (1, 0, 0)
  line L0 (0, 0) -> (0, -67.5)
  line L1 (0, -67.5) -> (67.5, -67.5)
  line L2 (0, -67.5) -> (-67.5, -67.5)
  circle A0 centre (-67.5, -67.5) radius 1.5
  circle A1 centre (67.5, -67.5) radius 1.5
  dimension "d462" = 67.5
  dimension "d463" = 67.5
  dimension "d464" = 67.5
  dimension "d465" = 3
  dimension "d466" = 3
  constraints: 6 end point, 2 centre point, 2 coincident, 2 horizontal, 1 vertical
  measures "d462" distance of L0.start L0.end
  measures "d463" distance of L0.end L1.end
  measures "d464" distance of L0.end L2.end
  measures "d465" diameter of A0
  measures "d466" diameter of A1
extrude "Extrusion20" cut sketch "Sketch28" against normal blind 3
sketch "Sketch29" plane through (0, 3, 0) normal (0, 1, 0) x (1, 0, 0)
  circle A0 centre (-93.6948, -25.1054) radius 1.5 projected
  circle A1 centre (-93.6948, -25.1054) radius 1.5
  circle A2 centre (93.6948, -25.1054) radius 1.5 projected
  circle A3 centre (93.6948, -25.1054) radius 1.5
  point P0 (0, 0)
  dimension "d469" = 3
  dimension "d470" = 3
  constraints: 2 centre point, 2 coincident
  measures "d469" diameter of A1
  measures "d470" diameter of A3
extrude "Extrusion21" add sketch "Sketch29" against normal blind 3
sketch "Sketch31" plane through (0, 3, 0) normal (0, 1, 0) x (1, 0, 0)
  circle A0 centre (-37.6149, 37.9983) radius 1.5 projected
  circle A1 centre (-51.7149, 13.5763) radius 1.5 projected
  line L0 (-37.6149, 37.9983) -> (-51.7149, 13.5763)
  line L1 (-44.6649, 25.7873) -> (-72.8107, 42.0373)
  line L2 (-44.6649, 25.7873) -> (-12.1649, 25.7873) construction
  line L3 (0, 0) -> (-72.8107, 42.0373)
  dimension "d475" = 32.5
  dimension "d476" = 150
  constraints: 8 end point, 1 coincident, 1 equal length, 1 horizontal, 1 midpoint
  measures "d475" distance of L1.start L1.end
  measures "d476" angle of L2 L1
body "Solid1"
